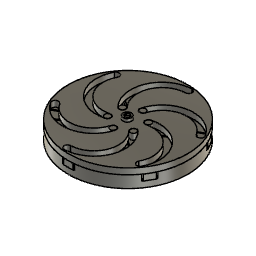
6 Pin Expanding Mechanism (Autodesk Fusion 360 design; units mm, degrees)
Autodesk Fusion 360 part; units mm, degrees
sketch "Sketch1" plane through (0, 0, 0) normal (0, 0, 1) x (1, 0, 0)
  circle A0 centre (0, 0) radius 50
  constraint coincident A0.centre origin
extrude "Extrude1" add sketch "Sketch1" along normal blind 5 makes body 1
sketch "Sketch2" plane through (0, 0, 5) normal (0, 0, 1) x (-1, 0, 0)
  circle A0 centre (0, 0) radius 50
  line L0 (5, 0) -> (-5, 0)
  line L1 (-5, 0) -> (-5, -54)
  line L2 (-5, -54) -> (5, -54)
  line L3 (5, -54) -> (5, 0)
  constraint horizontal L0
  constraint vertical L1
  constraint horizontal L2
  constraint vertical L3
extrude "Extrude2" add sketch "Sketch2" along normal blind 5 contours A0 L0 L1 L3 picked at (-1.0958, 16.6306) bodies 1
pattern_circular "C-Pattern1" count 6 over 360 about axis through (0, 0, 1.75) along (0, 0, 1) of 4 faces at (5, 16.5831, 6.6667) (0.5564, 16.6574, 5) (-5, 33.1662, 6.6667) (-1.6667, 0, 6.6667) on bodies 1
ref_plane "WorkPlane1" through (0, -0.1253, 15) normal (0, 0, 1) x (-1, 0, 0)
sketch "Sketch3" plane through (0, 0, 15) normal (0, 0, 1) x (1, 0, 0)
  line L0 (4, -10) -> (-4, -10)
  line L1 (-4, -10) -> (-4, -50)
  line L2 (-4, -50) -> (4, -50)
  line L3 (4, -50) -> (4, -10)
  circle A0 centre (0, -12.5) radius 2.5
  constraint horizontal L0
  constraint vertical L1
  constraint horizontal L2
  constraint vertical L3
extrude "Extrude3" add sketch "Sketch3" along normal blind 5 separate body makes body 2
extrude "Extrude4" add sketch "Sketch3" along normal blind 10 contours A0 bodies 2
pattern_circular "C-Pattern2" count 6 over 360 about axis through (0, 0, 1.75) along (0, 0, 1) of bodies 2 makes body 3 at (32.4209, -17.1786, 15) makes body 4 at (31.0876, 19.488, 15) makes body 5 at (-1.3333, 36.6667, 15) makes body 6 at (-32.4209, 17.1786, 15) makes body 7 at (-31.0876, -19.488, 15)
ref_plane "WorkPlane2" through (0, -12.5, 30) normal (0, 0, 1) x (1, 0, 0)
sketch "Sketch4" plane through (0, 0, 30) normal (0, 0, 1) x (1, 0, 0)
  circle A0 centre (0, 0) radius 50
  arc A1 (-39.8993, -17.2819) -> (-2.6497, -11.764) centre (-22.5, -6.25) ccw
  arc A2 (-44.5443, -20.227) -> (2.6497, -13.236) centre (-22.5, -6.25) ccw
  arc A3 (2.6497, -13.236) -> (-2.6497, -11.764) centre (0, -12.5) ccw
  arc A4 (-39.8993, -17.2819) -> (-44.5443, -20.227) centre (-42.2218, -18.7545) ccw
  dimension "d15" = 5.5
  constraint coincident A0.centre origin
  constraint tangent A1 A4
  measures "d15" diameter of A3
extrude "Extrude5" add sketch "Sketch4" along normal blind 5 separate body makes body 8
pattern_circular "C-Pattern3" count 6 over 360 about axis through (0, 0, 1.75) along (0, 0, 1) of 4 faces at (-31.0387, -30.9158, 33.3333) (-2.2381, -10.9021, 33.3333) (-4.531, -16.3274, 33.3333) (-41.6543, -16.0637, 33.3333) on bodies 8
hole "Hole1" at (0, 0, 35) direction (0, 0, -1) diameter 5 depth 80 tip angle 118 bodies 8 1
sketch "Sketch5" plane through (0, 0, 0) normal (0, 0, -1) x (1, 0, 0)
  circle A0 centre (0, 0) radius 2.5
  circle A1 centre (0, 0) radius 50
  line L0 (3.5, 2.0207) -> (0, 4.0415)
  line L1 (0, 4.0415) -> (-3.5, 2.0207)
  line L2 (-3.5, 2.0207) -> (-3.5, -2.0207)
  line L3 (-3.5, -2.0207) -> (0, -4.0415)
  line L4 (0, -4.0415) -> (3.5, -2.0207)
  line L5 (3.5, -2.0207) -> (3.5, 2.0207)
  dimension "d54" = 3.5
  constraint coincident A0.centre A1.centre
  measures "d54" distance of A0.centre L5
extrude "Extrude6" cut sketch "Sketch5" against normal blind 3 contours L0 L1 L2 L3 L4 L5 bodies 1
sketch "Sketch6" plane through (0, 0, 0) normal (0, 0, 1) x (1, 0, 0)
  circle A0 centre (90, 0) radius 3.5
  dimension "d57" = 7
  measures "d57" diameter of A0
extrude "Extrude7" add sketch "Sketch6" along normal blind 2.5 separate body makes body 9
sketch "Sketch7" plane through (0, 0, 2.5) normal (0, 0, 1) x (-1, 0, 0)
  circle A0 centre (-90, 0) radius 3.5
  circle A1 centre (-90, 0) radius 2.5
  dimension "d60" = 5
  constraint concentric A0 A1
  measures "d60" diameter of A1
extrude "Extrude8" add sketch "Sketch7" along normal blind 15 contours A1 bodies 9
thread "Thread1" "ISO Metric profile 5.0 M5x0.8 6g" major diameter 4.901 minor diameter 3.9895 pitch 0.8 angle 60 modelled right hand crest width 0.1157 on face at (87.5124, 0.2489, 12.5) from (90, 0, 7.5) to (90, 0, 17.5) crest through (87.5495, 0, 2.3) on bodies 9
sketch "Sketch8" plane through (0, 0, 0) normal (0, 0, -1) x (1, 0, 0)
  circle A0 centre (90, 0) radius 3.5
  line L0 (88, -1.1547) -> (90, -2.3094)
  line L1 (90, -2.3094) -> (92, -1.1547)
  line L2 (92, -1.1547) -> (92, 1.1547)
  line L3 (92, 1.1547) -> (90, 2.3094)
  line L4 (90, 2.3094) -> (88, 1.1547)
  line L5 (88, 1.1547) -> (88, -1.1547)
  point P0 (90, 0)
  constraint coincident P0 A0.centre
extrude "Extrude9" cut sketch "Sketch8" against normal blind 1.5 contours L0 L1 L2 L3 L4 L5 bodies 9
copy_body "Body->Comp9" bodies 9 removing the originals makes body 10 in component "Component''''''''"
copy_body "Body->Comp1" bodies 1 removing the originals makes body 11 in component "Component"
copy_body "Body->Comp2" bodies 2 removing the originals makes body 12 in component "Component'"
copy_body "Body->Comp3" bodies 3 removing the originals makes body 13 in component "Component''"
copy_body "Body->Comp4" bodies 4 removing the originals makes body 14 in component "Component'''"
copy_body "Body->Comp5" bodies 5 removing the originals makes body 15 in component "Component''''"
copy_body "Body->Comp6" bodies 6 removing the originals makes body 16 in component "Component'''''"
copy_body "Body->Comp7" bodies 7 removing the originals makes body 17 in component "Component''''''"
copy_body "Body->Comp8" bodies 8 removing the originals makes body 18 in component "Component'''''''"
move_body "Move1" bodies 14 to x (1, 0, 0) y (0, 1, 0) z (0, 0, 1) at (0, 0, -10) in component "Component'''"
move_body "Move1'" bodies 12 to x (1, 0, 0) y (0, 1, 0) z (0, 0, 1) at (0, 0, -10) in component "Component'"
move_body "Move1''" bodies 13 to x (1, 0, 0) y (0, 1, 0) z (0, 0, 1) at (0, 0, -10) in component "Component''"
move_body "Move1'''" bodies 15 to x (1, 0, 0) y (0, 1, 0) z (0, 0, 1) at (0, 0, -10) in component "Component''''"
move_body "Move1''''" bodies 16 to x (1, 0, 0) y (0, 1, 0) z (0, 0, 1) at (0, 0, -10) in component "Component'''''"
move_body "Move1'''''" bodies 17 to x (1, 0, 0) y (0, 1, 0) z (0, 0, 1) at (0, 0, -10) in component "Component''''''"
move_body "Move1''''''" bodies 10 to x (-1, 0, 0) y (0, 1, 0) z (0, 0, -1) at (89.4042, 0, 17.5) in component "Component''''''''"
component "Component" placed x (1, 0, 0) y (0, 1, 0) z (0, 0, 1) at (0, 0, 0)
component "Component'" placed x (1, 0, 0) y (0, 1, 0) z (0, 0, 1) at (0, 0, 0)
component "Component''" placed x (1, 0, 0) y (0, 1, 0) z (0, 0, 1) at (0, 0, 0)
component "Component'''" placed x (1, 0, 0) y (0, 1, 0) z (0, 0, 1) at (0, 0, 0)
component "Component''''" placed x (1, 0, 0) y (0, 1, 0) z (0, 0, 1) at (0, 0, 0)
component "Component'''''" placed x (1, 0, 0) y (0, 1, 0) z (0, 0, 1) at (0, 0, 0)
component "Component''''''" placed x (1, 0, 0) y (0, 1, 0) z (0, 0, 1) at (0, 0, 0)
component "Component'''''''" placed x (1, 0, 0) y (0, 1, 0) z (0, 0, 1) at (0, 0, -20)
component "Component''''''''" placed x (1, 0, 0) y (0, 1, 0) z (0, 0, 1) at (0, 0, 0)
